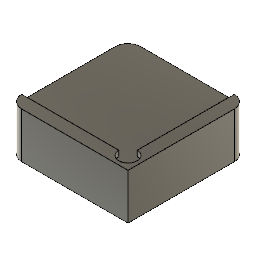
Corner Probe v2 (Autodesk Fusion 360 design; units mm, degrees)
Autodesk Fusion 360 part; units mm, degrees
sketch "Sketch1" plane through (0, 0, 0) normal (0, 0, 1) x (1, 0, 0)
  line L0 (0, 0) -> (-65, 0)
  line L1 (-65, 0) -> (-65, 65)
  line L2 (-65, 65) -> (0, 65)
  line L3 (0, 65) -> (0, 0)
  dimension "d1" = 65
  dimension "d2" = 65
  constraint horizontal L0
  constraint vertical L1
  constraint horizontal L2
  constraint vertical L3
  constraint coincident L0.start L3.end
  measures "d1" distance of L0.start L0.end
  measures "d2" distance of L0.start L2.end
extrude "Extrude1" add sketch "Sketch1" along normal blind 25
sketch "Sketch2" plane through (0, 0, 25) normal (0, 0, 1) x (-1, 0, 0)
  line L0 (0, -65) -> (65, -65)
  line L1 (65, -65) -> (65, 0)
  line L2 (65, 0) -> (0, 0)
  line L3 (0, 0) -> (0, -65)
  line L4 (0, 0) -> (65, 0)
  line L5 (65, 0) -> (65, -7)
  line L6 (65, -7) -> (0, -7)
  line L7 (0, -7) -> (0, 0)
  line L8 (0, 0) -> (7, 0)
  line L9 (7, 0) -> (7, -65)
  line L10 (7, -65) -> (0, -65)
  line L11 (0, -65) -> (0, 0)
  dimension "d5" = 65
  dimension "d6" = 7
  dimension "d7" = 7
  constraint horizontal L4
  constraint vertical L5
  constraint horizontal L6
  constraint vertical L7
  constraint coincident L2.end L3.start
  constraint horizontal L8
  constraint vertical L9
  constraint horizontal L10
  constraint vertical L11
  measures "d5" distance of L2.end L1.end
  measures "d6" distance of L2.end L6.end
  measures "d7" distance of L2.end L8.end
fillet "Fillet1" radius 7 1 edges at (-65, 0, 12.5)
fillet "Fillet2" radius 7 1 edges at (0, 65, 12.5)
fillet "Fillet3" radius 7 1 edges at (-65, 65, 12.5)
extrude "Extrude2" cut sketch "Sketch2" against normal blind 3 contours L0 L1 L6 L9
sketch "Sketch3" plane through (0, 0, 22) normal (0, 0, 1) x (-1, 0, 0)
  arc A0 (58, -65) -> (65, -58) centre (58, -58) ccw
  line L0 (65, -58) -> (65, -7)
  line L1 (65, -7) -> (7, -7)
  line L2 (7, -7) -> (7, -65)
  line L3 (7, -65) -> (58, -65)
  circle A1 centre (7, -7) radius 5
  dimension "d13" = 10
  constraint coincident L1.end L2.start
  measures "d13" diameter of A1
extrude "Extrude3" cut sketch "Sketch3" along normal blind 3 contours L1 L2 A1 | L1 L2 A1
sketch "Sketch4" plane through (0, 65, 0) normal (0, 1, 0) x (-1, 0, 0)
  line L0 (58, 22) -> (7, 22)
  line L1 (7, 22) -> (7, 0)
  line L2 (7, 0) -> (58, 0)
  line L3 (58, 0) -> (58, 22)
  circle A0 centre (32.6873, 10.9427) radius 2
  dimension "d16" = 4
  measures "d16" diameter of A0
extrude "Extrude4" cut sketch "Sketch4" against normal blind 25 contours A0
